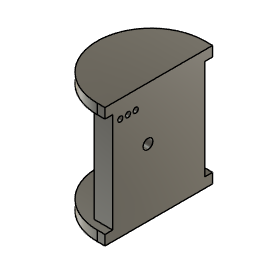
Tilt Plate v4 (Autodesk Fusion 360 design; units mm, degrees)
Autodesk Fusion 360 part; units mm, degrees
sketch "circle r" plane through (0, 0, 0) normal (0, 0, 1) x (1, 0, 0)
  line L0 (35.0001, 0) -> (-20.9999, 0)
  arc A0 (14, 35) -> (14, -35) centre (14.0001, 0) ccw
  line L1 (14, 35) -> (14, -35)
  line L2 (35.0001, 0) -> (14.0001, 0)
  line L3 (0, -32.078) -> (0, 32.078)
  arc A1 (2.8227, 16.8933) -> (-2.8225, 16.8952) centre (0, 16.5) ccw
  line L4 (2.8225, -16.8952) -> (4.6322, -3.969)
  circle A2 centre (0, 0) radius 4.55
  arc A3 (-4.6322, 3.969) -> (-4.6322, -3.969) centre (0, 0) ccw
  line L5 (-4.6322, -3.969) -> (-2.8225, -16.8952)
  arc A4 (-2.8225, -16.8952) -> (2.8225, -16.8952) centre (0, -16.5) ccw
  arc A5 (4.6322, -3.969) -> (4.6322, 3.969) centre (0, 0) ccw
  line L6 (2.8225, 16.8952) -> (4.6322, 3.969)
  line L7 (-4.6322, 3.969) -> (-2.8225, 16.8952)
  point P0 (0, -32.078)
  point P1 (6.1, 0)
  dimension "d38" = 35
  dimension "d39" = 70
  dimension "d40" = 14
  dimension "d49" = 56
  dimension "d93" = 9.1
  dimension "d94" = 6.1
  dimension "d95" = 2.85
  dimension "d96" = 33.7903
  dimension "d98" = 7.938
  dimension "d99" = 12.9262
  constraint horizontal L0
  constraint coincident L0.end A0
  constraint vertical A0.start A0.end
  constraint coincident A2.centre L0
  constraint coincident L0 A0.centre
  constraint coincident L0 L2.start
  constraint coincident A0.centre L2.end
  constraint coincident P0 A0
  constraint coincident P0 L3.start
  constraint coincident A0 L3.end
  constraint coincident A2.centre L3
  constraint vertical L3
  constraint tangent L4 A4
  constraint tangent L5 A4
  constraint midpoint P1 A5
  constraint symmetric L3 L4 L5
  constraint symmetric L3 A3 A5
  constraint coincident A2.centre A3.centre
  constraint coincident L3 A2.centre
  constraint symmetric L0 L4.end A5.end
  constraint symmetric L0 L4.start L6.start
  constraint coincident A5.end L6
  constraint coincident A1.end L7
  constraint coincident A1 L7.end
  constraint coincident A1 L6.start
  constraint coincident A1.start L6
  constraint coincident A3 L7.start
  constraint coincident A3.start L7
  constraint symmetric L0 L5 L7
  constraint symmetric L0 A1 A4
  constraint coincident L0 A2.centre
  constraint coincident L0.start L2.start
  measures "d38" radius of A0
  measures "d39" distance of A0.start A0.end
  measures "d40" distance of P0 L1
  measures "d49" distance of L0.start L0.end
  measures "d93" diameter of A2
  measures "d94" radius of A3
  measures "d95" radius of A1
  measures "d96" distance of A1.end L5.end
  measures "d98" distance of L4.end A5.end
  measures "d99" vertical distance of A3.end L5.end
extrude "Extrude1" add sketch "circle r" along normal blind 6.5 contours L0 A0 L1 L3 L4 A4 A5 | L0 A0 L1 L3 A1 A5 L6 | L0 A0 L3 A1 A3 L7 | L0 A0 L3 A3 L5 A4
extrude "Extrude2" add sketch "circle r" along normal blind 3.5 contours L0 L3 L4 A2 A4 A5 | L0 L3 A1 A2 A5 L6 | L0 L3 A1 A2 A3 L7 | L0 L3 A2 A3 L5 A4
sketch "platform" plane through (0, 0, 6.5) normal (0, 0, 1) x (-1, 0, 0)
  line L0 (-14, -30) -> (-7, -30)
  line L1 (-7, -30) -> (-7, 30)
  line L2 (-7, 30) -> (-14, 30)
  line L3 (-14, 30) -> (-14, -30)
  line L4 (-14, 0) -> (20.9999, 0)
  arc A0 (-14, -35) -> (-14, 35) centre (-14.0001, 0) ccw
  line L5 (-14, 35) -> (-14, -35)
  dimension "d51" = 60
  dimension "d83" = 7
  constraint horizontal L0
  constraint vertical L1
  constraint horizontal L2
  constraint vertical L3
  constraint midpoint L3 L4.start
  constraint perpendicular L1 L4
  constraint coincident L4.end A0
  constraint coincident L2.end L5
  constraint coincident L4 A0.centre
  measures "d51" distance of L0.start L2.end
  measures "d83" distance of L0.start L0.end
extrude "Extrude5" add sketch "platform" along normal blind 65 contours L0 L1 L3 L4 L5 | L1 L2 L3 L4 L5
sketch "circle l" plane through (0, 0, 71.5) normal (0, 0, 1) x (-1, 0, 0)
  arc A0 (-14, -35) -> (-14, 35) centre (-14, 0) ccw
  line L0 (-14, -35) -> (-14, 35)
  line L1 (-14, 30) -> (-14, -30)
  point P0 (-14, -35)
  point P1 (-14, 35)
  point P2 (-14, 35)
  point P3 (-14, -35)
  dimension "d43" = 35
  constraint coincident A0.centre L0
  constraint coincident P3 P0
  constraint coincident P1 A0.end
  measures "d43" radius of A0
extrude "Extrude9" add sketch "circle l" along normal blind 6.5
sketch "camera hole" plane through (14, 0, 0) normal (1, 0, 0) x (0, 1, 0)
  line L0 (0, 78) -> (0, 0)
  line L1 (30, 39) -> (-30, 39)
  line L2 (30, 6.5) -> (30, 71.5)
  line L3 (-30, 6.5) -> (-30, 71.5)
  line L4 (-35, 78) -> (35, 78)
  line L5 (-3.775, 6.5) -> (-3.775, 78) construction
  line L6 (-30, 6.5) -> (30, 6.5)
  circle A0 centre (-7, 43.5) radius 3.225
  line L7 (-30, 71.5) -> (-35, 71.5)
  line L8 (35, 71.5) -> (30, 71.5)
  line L9 (35, 0) -> (35, 6.5)
  line L10 (35, 6.5) -> (30, 6.5)
  line L11 (30, 6.5) -> (30, 71.5)
  line L12 (30, 71.5) -> (35, 71.5)
  line L13 (35, 71.5) -> (35, 78)
  line L14 (35, 78) -> (-35, 78)
  line L15 (-35, 78) -> (-35, 71.5)
  line L16 (-35, 71.5) -> (-30, 71.5)
  line L17 (-30, 71.5) -> (-30, 6.5)
  line L18 (-30, 6.5) -> (-35, 6.5)
  line L19 (-35, 6.5) -> (-35, 0)
  line L20 (-35, 0) -> (35, 0)
  point P0 (-3.775, 43.5)
  dimension "d68" = 6.45
  dimension "d74" = 7
  dimension "d81" = 9
  constraint coincident L0.end origin
  constraint vertical L0
  constraint horizontal L1
  constraint midpoint L1.start L2
  constraint coincident L1.end L3
  constraint coincident L0.start L4
  constraint perpendicular L1 L5
  constraint coincident L5.start L6
  constraint coincident A0 P0
  constraint coincident L5 P0
  constraint horizontal A0.centre P0
  constraint coincident L4 L5.end
  measures "d68" diameter of A0
  measures "d74" distance of L0 A0.centre
extrude "Extrude11" cut sketch "camera hole" against normal blind 10 contours A0
sketch "linear actuator hole" plane through (14, 0, 0) normal (1, 0, 0) x (0, 1, 0)
  circle A0 centre (-25, 66.5) radius 1.675
  line L0 (30, 6.5) -> (30, 71.5)
  circle A1 centre (-7, 43.5) radius 3.225
  line L1 (-30, 71.5) -> (-30, 6.5)
  line L2 (-30, 6.5) -> (-30, 71.5)
  circle A2 centre (-20, 66.5) radius 1.675
  circle A3 centre (-15, 66.5) radius 1.675
  line L3 (30, 71.5) -> (35, 71.5)
  line L4 (35, 0) -> (35, 6.5)
  line L5 (35, 6.5) -> (30, 6.5)
  line L6 (35, 71.5) -> (35, 78)
  line L7 (35, 78) -> (-35, 78)
  line L8 (-35, 78) -> (-35, 71.5)
  line L9 (-35, 71.5) -> (-30, 71.5)
  line L10 (-30, 6.5) -> (-35, 6.5)
  line L11 (-35, 6.5) -> (-35, 0)
  line L12 (-35, 0) -> (35, 0)
  dimension "d55" = 3.35
  dimension "d71" = 5
  dimension "d77" = 10
  dimension "d78" = 0
  dimension "d91" = 5
  measures "d55" diameter of A0
  measures "d71" distance of A0.centre L2
  measures "d91" distance of A0.centre L9
extrude "Extrude12" cut sketch "linear actuator hole" against normal blind 13 contours A0 | A2 | A3
sketch "connector hole" plane through (0, 0, 71.5) normal (0, 0, -1) x (1, 0, 0)
  arc A0 (14, 35) -> (14, -35) centre (14, 0) ccw
  line L0 (14, 30) -> (14, 35)
  circle A1 centre (3, 0) radius 1.675
  line L1 (7, -30) -> (7, 30)
  line L2 (7, 30) -> (14, 30)
  line L3 (14, -35) -> (14, -30)
  line L4 (14, -30) -> (7, -30)
  line L5 (7, -30) -> (7, 30)
  line L6 (7, 30) -> (14, 30)
  line L7 (14, 30) -> (14, 35)
  arc A2 (14, 35) -> (14, -35) centre (14, 0) ccw
  line L8 (14, -35) -> (14, -30)
  line L9 (14, -30) -> (7, -30)
  line L10 (7, -30) -> (7, 30)
  dimension "d60" = 3.35
  dimension "d61" = 4
  constraint horizontal origin A1.centre
  measures "d60" diameter of A1
  measures "d61" distance of A1.centre L1
extrude "Extrude14" add 2 faces at (14, 18.7297, 40.3398) (14, -10, 2.1667) along direction (1, 0, 0) blind 5
